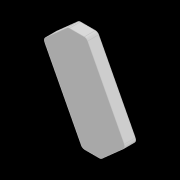
# Autodesk Inventor part: switchback-pickup-cover-6
Saved by Autodesk Inventor 2020 (Build 240168000, 168)
## iProperties
Created: 2020-01-09
Part Number: switchback-pickup-cover-6
Material: Generic
Document SubType Name: Modeling
Designer: valer
Density: 1 g/cm^3
Appearance: Default
Author: valer
Autodesk Inventor part; units mm, degrees
ref_plane "YZ Plane" through (0, 0, 0) normal (1, 0, 0) x (0, 1, 0)
ref_plane "XZ Plane" through (0, 0, 0) normal (0, 1, 0) x (-1, 0, 0)
ref_plane "XY Plane" through (0, 0, 0) normal (0, 0, 1) x (1, 0, 0)
sketch "TopProfile" plane through (0, 0, 0) normal (0, 0, 1) x (1, 0, 0)
  line L0 (-12.5751, 79.2329) -> (-31.9912, 61.979)
  line L1 (1.4359, 79.2329) -> (-31.9912, 61.979) construction
  line L2 (-12.5751, 79.2329) -> (1.4359, 79.2329)
  line L3 (-31.9912, 61.979) -> (0, 0)
  line L4 (1.4359, 79.2329) -> (33.4272, 17.2538)
  line L5 (0, 0) -> (33.4272, 17.2538) construction
  line L6 (14.011, 0) -> (33.4272, 17.2538)
  line L7 (0, 0) -> (14.011, 0)
  line L8 (-48.1736, 0) -> (49.6096, 0) construction
  line L9 (-10.7561, 72.9398) -> (-8.499, 74.1048)
  line L10 (-8.499, 74.1048) -> (-11.4466, 79.8154)
  line L11 (-11.4466, 79.8154) -> (-13.7036, 78.6504)
  line L12 (-13.7036, 78.6504) -> (-10.7561, 72.9398)
  line L13 (9.9349, 5.128) -> (12.192, 6.293)
  line L14 (12.192, 6.293) -> (15.1396, 0.5825)
  line L15 (15.1396, 0.5825) -> (12.8825, -0.5825)
  line L16 (12.8825, -0.5825) -> (9.9349, 5.128)
  line L17 (35.6405, 16.8421) -> (14.6869, -1.778)
  line L18 (14.6869, -1.778) -> (-1.0831, -1.778)
  line L19 (-1.0831, -1.778) -> (-34.2046, 62.3907)
  line L20 (-34.2046, 62.3907) -> (-13.2509, 81.0109)
  line L21 (-13.2509, 81.0109) -> (2.5191, 81.0109)
  line L22 (2.5191, 81.0109) -> (35.6405, 16.8421)
  point P0 (-11.1459, 79.2329)
  point P1 (-13.5549, 78.3622)
  point P2 (14.9908, 0.8707)
  point P3 (12.5818, 0)
  dimension "d0" = 37.6174
  dimension "d1" = 165.676
  dimension "d2" = 19.4161
  dimension "d3" = 69.7484
  dimension "d4" = 62.699
  dimension "d5" = 37.6174
  dimension "d6" = 165.676
  dimension "d15" = 2.54
  dimension "d16" = 1.778
  constraints: 46 end point, 6 parallel, 3 perpendicular, 2 collinear, 2 horizontal, 2 midpoint, 2 point on line, 5 other
  measures "d0" distance between parallel lines of L3 L4
  measures "d1" angle of L1 L0
  measures "d2" horizontal distance of L2.start L0.end
  measures "d3" distance of L3.end L0.end
  measures "d4" angle of L8 L3
  measures "d5" distance of L1.start L1.end
  measures "d6" angle of L5 L6
  measures "d15" distance of L10.end L11.end
  measures "d16" distance between parallel lines of L4 L22
extrude "CapFeature" add sketch "TopProfile" along normal blind 1.778 contours L2 L10 L9 L12 L0 | L11 L10 L2 | L0 L12 L11 | L12 L9 L10 L2 L4 L6 L14 L13 L16 L7 L3 L0 | L16 L13 L14 L6 L7 | L7 L15 L16 | L14 L15 L6 | L17 L18 L19 L20 L21 L22
extrude "WallsFeature" add sketch "TopProfile" against normal blind 7.62 contours L2 L10 L9 L12 L0 | L11 L10 L2 | L0 L12 L11 | L16 L13 L14 L6 L7 | L7 L15 L16 | L14 L15 L6 | L17 L18 L19 L20 L21 L22
fillet "SideFilletsFeature" radius 3.175 10 edges at (-31.9912, 61.979, -3.81) (0, 0, -3.81) (33.4272, 17.2538, -3.81) (1.4359, 79.2329, -3.81) (2.5191, 81.0109, -2.921) (-13.2509, 81.0109, -2.921) (-34.2046, 62.3907, -2.921) (35.6405, 16.8421, -2.921) (14.6869, -1.778, -2.921) (-1.0831, -1.778, -2.921)
body "Solid1"
